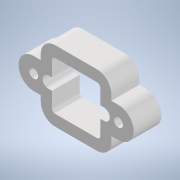
# Autodesk Inventor part: ramka
Saved by Autodesk Inventor 2020 (Build 240168000, 168)
## iProperties
Created: 2022-10-14
Part Number: ramka
Material: Типовые
Document SubType Name: Modeling
Designer: akapu
Density: 1 g/cm^3
Appearance: По умолчанию
Author: akapu
Autodesk Inventor part; units mm, degrees
ref_plane "YZ Plane" through (0, 0, 0) normal (1, 0, 0) x (0, 1, 0)
ref_plane "XZ Plane" through (0, 0, 0) normal (0, 1, 0) x (-1, 0, 0)
ref_plane "XY Plane" through (0, 0, 0) normal (0, 0, 1) x (1, 0, 0)
sketch "Эскиз1" plane through (0, 0, 0) normal (0, 0, 1) x (1, 0, 0)
  line L0 (16.51, 16.51) -> (0, 16.51) projected
  line L1 (0, 16.51) -> (0, 11.176) projected
  line L2 (0, 11.176) -> (-6.731, 11.176) projected
  line L3 (-6.731, 11.176) -> (-7.4684, 11.0622) projected
  line L4 (-7.4684, 11.0622) -> (-8.1512, 10.7614) projected
  line L5 (-8.1512, 10.7614) -> (-8.733, 10.2942) projected
  line L6 (-8.733, 10.2942) -> (-9.1739, 9.6923) projected
  line L7 (-9.1739, 9.6923) -> (-9.4441, 8.9967) projected
  line L8 (-9.4441, 8.9967) -> (-9.525, 8.255) projected
  line L9 (-9.525, 8.255) -> (-9.4441, 7.5133) projected
  line L10 (-9.4441, 7.5133) -> (-9.1739, 6.8177) projected
  line L11 (-9.1739, 6.8177) -> (-8.733, 6.2158) projected
  line L12 (-8.733, 6.2158) -> (-8.1512, 5.7486) projected
  line L13 (-8.1512, 5.7486) -> (-7.4684, 5.4478) projected
  line L14 (-7.4684, 5.4478) -> (-6.731, 5.334) projected
  line L15 (-6.731, 5.334) -> (0, 5.334) projected
  line L16 (0, 5.334) -> (0, 0) projected
  line L17 (0, 0) -> (16.51, 0) projected
  line L18 (16.51, 0) -> (16.51, 5.334) projected
  line L19 (16.51, 5.334) -> (23.241, 5.334) projected
  line L20 (23.241, 5.334) -> (23.9784, 5.4478) projected
  line L21 (23.9784, 5.4478) -> (24.6612, 5.7486) projected
  line L22 (24.6612, 5.7486) -> (25.243, 6.2158) projected
  line L23 (25.243, 6.2158) -> (25.6839, 6.8177) projected
  line L24 (25.6839, 6.8177) -> (25.9541, 7.5133) projected
  line L25 (25.9541, 7.5133) -> (26.035, 8.255) projected
  line L26 (26.035, 8.255) -> (25.9541, 8.9967) projected
  line L27 (25.9541, 8.9967) -> (25.6839, 9.6923) projected
  line L28 (25.6839, 9.6923) -> (25.243, 10.2942) projected
  line L29 (25.243, 10.2942) -> (24.6612, 10.7614) projected
  line L30 (24.6612, 10.7614) -> (23.9784, 11.0622) projected
  line L31 (23.9784, 11.0622) -> (23.241, 11.176) projected
  line L32 (23.241, 11.176) -> (16.51, 11.176) projected
  line L33 (16.51, 11.176) -> (16.51, 16.51) projected
  circle A0 centre (18.26, 8.26) radius 1.27 projected
  circle A1 centre (-1.75, 8.26) radius 1.27 projected
  circle A2 centre (11.505, 9.45) radius 0.127 projected
  circle A3 centre (8.386, 9.267) radius 0.127 projected
  circle A4 centre (4.826, 15.748) radius 0.127 projected
  circle A5 centre (4.191, 15.748) radius 0.127 projected
  circle A6 centre (-6.985, 8.255) radius 1.5 projected
  circle A7 centre (23.495, 8.255) radius 1.5 projected
  circle A8 centre (3.048, 4.445) radius 0.1651 projected
  circle A9 centre (6.985, 4.445) radius 0.1651 projected
  circle A10 centre (2.286, 6.731) radius 0.2032 projected
  circle A11 centre (13.716, 8.509) radius 0.2032 projected
  circle A12 centre (12.319, 1.778) radius 0.2032 projected
  circle A13 centre (15.367, 16.002) radius 0.2032 projected
  circle A14 centre (14.732, 1.778) radius 0.2032 projected
  circle A15 centre (13.462, 1.778) radius 0.2032 projected
  circle A16 centre (11.5062, 15.748) radius 0.127 projected
  circle A17 centre (7.874, 15.748) radius 0.127 projected
  circle A18 centre (3.429, 14.859) radius 0.127 projected
  circle A19 centre (14.478, 15.113) radius 0.1651 projected
  circle A20 centre (2.286, 10.541) radius 0.2032 projected
  circle A21 centre (13.716, 11.176) radius 0.2032 projected
  circle A22 centre (5.505, 15.748) radius 0.127 projected
  circle A23 centre (14.478, 14.224) radius 0.1651 projected
  circle A24 centre (13.462, 15.113) radius 0.1651 projected
  circle A25 centre (10.414, 15.7988) radius 0.127 projected
  circle A26 centre (5.005, 9.727) radius 0.127 projected
  circle A27 centre (6.8072, 8.636) radius 0.127 projected
  circle A28 centre (4.699, 8.382) radius 0.127 projected
  circle A29 centre (10.922, 8.636) radius 0.127 projected
  circle A30 centre (6.378, 16.129) radius 0.127 projected
  circle A31 centre (10.4648, 5.4864) radius 0.127 projected
  circle A32 centre (11.2268, 5.4864) radius 0.127 projected
  circle A33 centre (10.4648, 6.1214) radius 0.127 projected
  circle A34 centre (9.1948, 7.8994) radius 0.127 projected
  circle A35 centre (2.955, 14.2) radius 0.3 projected
  circle A36 centre (9.779, 15.748) radius 0.127 projected
  circle A37 centre (9.906, 8.636) radius 0.127 projected
  circle A38 centre (9.194, 7.112) radius 0.127 projected
  circle A39 centre (9.144, 15.748) radius 0.127 projected
  circle A40 centre (5.588, 7.874) radius 0.127 projected
  circle A41 centre (13.335, 6.096) radius 0.1651 projected
  circle A42 centre (6.8072, 7.874) radius 0.127 projected
  circle A43 centre (6.878, 15.748) radius 0.127 projected
  circle A44 centre (7.378, 16.141) radius 0.127 projected
  circle A45 centre (5.588, 7.239) radius 0.127 projected
  circle A46 centre (8.509, 15.748) radius 0.127 projected
  circle A47 centre (7.5946, 7.1186) radius 0.127 projected
  circle A48 centre (13.555, 14.2) radius 0.3 projected
  line L34 (9.655, 16.755) -> (9.655, 15.8775) projected
  arc A49 (6.855, 15.8775) -> (9.655, 15.8775) centre (8.255, 8.255) ccw projected
  line L35 (6.855, 15.8775) -> (6.855, 16.755) projected
  line L36 (6.855, 16.755) -> (0.755, 16.755) projected
  arc A50 (0.755, 16.755) -> (-0.245, 15.755) centre (0.755, 15.755) ccw projected
  line L37 (-0.245, 15.755) -> (-0.245, 10.155) projected
  line L38 (-0.245, 10.155) -> (-1.745, 10.155) projected
  arc A51 (-1.745, 10.155) -> (-1.745, 6.355) centre (-1.745, 8.255) ccw projected
  line L39 (-1.745, 6.355) -> (-0.245, 6.355) projected
  line L40 (-0.245, 6.355) -> (-0.245, 0.755) projected
  arc A52 (-0.245, 0.755) -> (0.755, -0.245) centre (0.755, 0.755) ccw projected
  line L41 (0.755, -0.245) -> (15.755, -0.245) projected
  arc A53 (15.755, -0.245) -> (16.755, 0.755) centre (15.755, 0.755) ccw projected
  line L42 (16.755, 0.755) -> (16.755, 6.355) projected
  line L43 (16.755, 6.355) -> (18.255, 6.355) projected
  arc A54 (18.255, 6.355) -> (18.255, 10.155) centre (18.255, 8.255) ccw projected
  line L44 (18.255, 10.155) -> (16.755, 10.155) projected
  line L45 (16.755, 10.155) -> (16.755, 15.755) projected
  arc A55 (16.755, 15.755) -> (15.755, 16.755) centre (15.755, 15.755) ccw projected
  line L46 (15.755, 16.755) -> (9.655, 16.755) projected
  circle A56 centre (-1.745, 8.255) radius 0.9 projected
  circle A57 centre (18.255, 8.255) radius 0.9 projected
  line L47 (-1.745, 10.355) -> (-0.445, 10.355)
  line L48 (-0.445, 10.355) -> (-0.445, 15.755)
  arc A58 (0.755, 16.955) -> (-0.445, 15.755) centre (0.755, 15.755) ccw
  line L49 (0.755, 16.955) -> (7.055, 16.955)
  line L50 (7.055, 16.955) -> (7.055, 15.709)
  arc A59 (7.055, 15.709) -> (9.455, 15.709) centre (8.255, 8.255) ccw
  line L51 (9.455, 15.709) -> (9.455, 16.955)
  line L52 (9.455, 16.955) -> (15.755, 16.955)
  arc A60 (16.955, 15.755) -> (15.755, 16.955) centre (15.755, 15.755) ccw
  line L53 (16.955, 15.755) -> (16.955, 10.355)
  line L54 (16.955, 10.355) -> (18.255, 10.355)
  arc A61 (18.255, 6.155) -> (18.255, 10.355) centre (18.255, 8.255) ccw
  line L55 (18.255, 6.155) -> (16.955, 6.155)
  line L56 (16.955, 6.155) -> (16.955, 0.755)
  arc A62 (15.755, -0.445) -> (16.955, 0.755) centre (15.755, 0.755) ccw
  line L57 (15.755, -0.445) -> (0.755, -0.445)
  arc A63 (-0.445, 0.755) -> (0.755, -0.445) centre (0.755, 0.755) ccw
  line L58 (-0.445, 0.755) -> (-0.445, 6.155)
  line L59 (-0.445, 6.155) -> (-1.745, 6.155)
  arc A64 (-1.745, 10.355) -> (-1.745, 6.155) centre (-1.745, 8.255) ccw
  line L60 (7.055, 16.955) -> (9.455, 16.955)
  line L61 (7.055, 20.955) -> (0.755, 20.955)
  arc A65 (0.755, 20.955) -> (-4.445, 15.755) centre (0.755, 15.755) ccw
  line L62 (-4.445, 15.755) -> (-4.445, 13.7249)
  line L63 (-4.445, 2.7851) -> (-4.445, 0.755)
  line L64 (20.955, 0.755) -> (20.955, 2.7851)
  line L65 (20.955, 13.7249) -> (20.955, 15.755)
  arc A66 (20.955, 15.755) -> (15.755, 20.955) centre (15.755, 15.755) ccw
  line L66 (15.755, 20.955) -> (9.455, 20.955)
  line L67 (7.055, 20.955) -> (9.455, 20.955)
  circle A67 centre (23.495, 8.255) radius 5.4699
  circle A68 centre (-6.985, 8.255) radius 5.4699
  line L68 (-6.985, 13.7249) -> (-4.445, 13.7249)
  line L69 (-4.445, 2.7851) -> (-6.985, 2.7851)
  line L70 (20.955, 2.7851) -> (23.495, 2.7851)
  line L71 (20.955, 13.7249) -> (23.495, 13.7249)
  circle A69 centre (-6.985, 8.255) radius 1.6
  circle A70 centre (23.495, 8.255) radius 1.6
  line L72 (-4.445, 0.755) -> (20.955, 0.755)
  line L73 (20.955, -5.445) -> (-4.445, -5.445)
  line L74 (28.9649, 8.255) -> (28.9649, -5.445)
  line L75 (28.9649, -5.445) -> (-12.4549, -5.445)
  line L76 (-12.4549, -5.445) -> (-12.4549, 8.255)
  point P0 (-0.445, 0.755)
  point P1 (-4.445, -5.445)
  dimension "d0" = 0.2
  dimension "d1" = 4
  dimension "d2" = 3.2
  dimension "d3" = 3.2
  constraints: 60 end point, 21 point on circle, 12 centre point, 4 coincident, 3 horizontal, 2 collinear, 2 parallel, 2 point on line, 2 tangent, 26 other
  measures "d0" distance between parallel lines of L38 L47
  measures "d1" distance between parallel lines of L53 L65
  measures "d2" diameter of A69
  measures "d3" diameter of A70
extrude "Выдавливание1" add sketch "Эскиз1" along normal blind 10 contours L60 L49 A58 L48 L2 A68 L68 L62 A65 L61 L67 L66 A66 L65 L71 A67 L32 L53 A60 L52 | L32 A67 A61 L54 L53 | A67 L19 L20 L21 L22 L23 L24 L25 L26 L27 L28 L29 L30 L31 L32 | L32 L31 L30 L29 L28 L27 L26 L25 L24 L23 L22 L21 L20 L19 A67 A61 | L74 L75 L73 L76 A68 L69 L63 L72 A63 L57 A62 L64 L70 A67 | A67 L19 L56 L55 A61 | L48 L47 A64 A68 L2 | L70 L64 L72 L56 L19 A67 | A68 A64 L15 L14 L13 L12 L11 L10 L9 L8 L7 L6 L5 L4 L3 L2 | L2 L3 L4 L5 L6 L7 L8 L9 L10 L11 L12 L13 L14 L15 A68 | A64 L59 L58 L15 A68 | L72 L63 L69 A68 L15 L58
sketch "Эскиз3" plane through (-12.4549, -5.445, 0) normal (-1, 0, 0) x (0, 0, 1)
  line L0 (0, 0) -> (0, 13.7) projected
  line L1 (0, 5) -> (10, 5) projected
  line L2 (0, 0) -> (10, 0)
  line L3 (10, 0) -> (10, 5)
  line L4 (10, 5) -> (0, 5)
  line L5 (0, 5) -> (0, 0)
  line L6 (5, 5) -> (5, 0)
  line L7 (0, 0) -> (10, 0) projected
  circle A0 centre (5, 2.5) radius 1.6
  circle A1 centre (5, 2.5) radius 5
  line L8 (10, 0) -> (10, 13.7) projected
  point P0 (0, 5.445)
  point P1 (0.6699, 0)
  point P2 (0, 2.5)
  point P3 (10, 2.5)
  point P4 (9.3301, 0)
  dimension "d11" = 3.2
  constraints: 10 end point, 3 midpoint, 2 centre point, 2 parallel, 1 coincident, 1 horizontal, 1 perpendicular, 1 tangent
  measures "d11" diameter of A0
extrude "Выдавливание3" cut sketch "Эскиз3" against normal up to surface (41.4198 mm away) contours L0 A1 L2 | A1 L3 L2 | A0 L6 | L6 A0
sketch "Эскиз4" plane through (-12.4549, -5.445, 0) normal (-1, 0, 0) x (0, 0, 1)
  circle A0 centre (5, 2.5) radius 1.6 projected
  circle A1 centre (5, 2.5) radius 5
  line L0 (10, 0) -> (10, 13.7) projected
  arc A2 (0, 2.5) -> (0.6699, 0) centre (5, 2.5) ccw projected
  line L1 (0.6699, 0) -> (9.3301, 0) projected
  line L2 (0.6699, 0) -> (9.3301, 0)
  point P0 (0, 5.445)
  constraints: 2 end point, 1 centre point, 1 coincident, 1 collinear, 1 tangent
extrude "Выдавливание4" add sketch "Эскиз4" against normal up to surface (41.4198 mm away) contours A1 L1 picked at (4.43, -1.3536)
sketch "Эскиз5" plane through (28.9649, 8.255, 10) normal (1, 0, 0) x (0, 0, -1)
  line L0 (5, -11.2) -> (5, -8.5)
  line L1 (6.5588, -8.5) -> (8.1177, -11.2)
  line L2 (8.1177, -11.2) -> (6.5588, -13.9)
  line L3 (6.5588, -13.9) -> (3.4412, -13.9)
  line L4 (3.4412, -13.9) -> (1.8823, -11.2)
  line L5 (1.8823, -11.2) -> (3.4412, -8.5)
  line L6 (3.4412, -8.5) -> (6.5588, -8.5)
  dimension "d17" = 2.7
  constraints: 14 end point, 1 coincident, 1 midpoint, 1 vertical, 13 other
  measures "d17" distance of L0.start L0.end
extrude "Выдавливание5" cut sketch "Эскиз5" against normal blind 3
